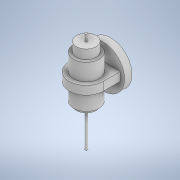
# Autodesk Inventor part: spindle
Saved by Autodesk Inventor 2020 (Build 240168000, 168)
## iProperties
Created: 2021-09-22
Part Number: spindle
Material: Generic
Document SubType Name: Modeling
Designer: zhang
Density: 1 g/cm^3
Appearance: Default
Author: zhang
Autodesk Inventor part; units mm, degrees
ref_plane "YZ Plane" through (0, 0, 0) normal (1, 0, 0) x (0, 1, 0)
ref_plane "XZ Plane" through (0, 0, 0) normal (0, 1, 0) x (-1, 0, 0)
ref_plane "XY Plane" through (0, 0, 0) normal (0, 0, 1) x (1, 0, 0)
sketch "Sketch1" plane through (0, 0, 0) normal (1, 0, 0) x (0, 1, 0)
  line L0 (0, 0) -> (1.5, 2)
  line L1 (1.5, 2) -> (1.5, 43)
  line L2 (0, 59) -> (0, 0)
  line L3 (11.5, 51) -> (16.5, 51)
  line L4 (16.5, 51) -> (16.5, 101)
  line L5 (16.5, 101) -> (11.5, 101)
  line L6 (1.5, 105) -> (1.5, 120)
  line L7 (1.5, 120) -> (0, 120)
  line L8 (0, 120) -> (0, 59)
  line L9 (0, -24) -> (0, 144) projected
  line L10 (16.5, 76) -> (-5.6648, 76)
  line L11 (-30.7978, 0) -> (145.133, 0) projected
  line L12 (11.5, 101) -> (11.5, 105)
  line L13 (11.5, 105) -> (1.5, 105)
  line L14 (11.5, 51) -> (11.5, 47)
  line L15 (11.5, 47) -> (5.5, 47)
  line L16 (5.5, 47) -> (5.5, 43)
  line L17 (5.5, 43) -> (1.5, 43)
  line L18 (0, 0) -> (2, 1.5)
  line L19 (2, 1.5) -> (43, 1.5)
  line L20 (43, 1.5) -> (43, 5.5)
  line L21 (43, 5.5) -> (47, 5.5)
  line L22 (47, 5.5) -> (47, 11.5)
  line L23 (47, 11.5) -> (51, 11.5)
  line L24 (51, 11.5) -> (51, 15)
  line L25 (51, 15) -> (101, 15)
  line L26 (101, 15) -> (101, 11.5)
  line L27 (101, 11.5) -> (112, 11.5)
  line L28 (112, 11.5) -> (112, 1.5)
  line L29 (112, 1.5) -> (120, 1.5)
  line L30 (120, 1.5) -> (120, 0)
  line L31 (-30.7978, 0) -> (145.133, 0) projected
  line L32 (76, 15) -> (76, 0)
  line L33 (0, 0) -> (120, 0)
  dimension "d0" = 2
  dimension "d3" = 76
  dimension "d4" = 120
  dimension "d5" = 50
  dimension "d7" = 1.5
  dimension "d8" = 10
  dimension "d9" = 4
  dimension "d10" = 4
  dimension "d11" = 4
  dimension "d12" = 6
  dimension "d13" = 4
  dimension "d21" = 2
  dimension "d22" = 1.5
  dimension "d23" = 76
  dimension "d24" = 120
  dimension "d25" = 1.5
  dimension "d26" = 4
  dimension "d27" = 4
  dimension "d28" = 6
  dimension "d29" = 4
  dimension "d30" = 10
  dimension "d31" = 8
  dimension "d32" = 50
  dimension "d33" = 15
  dimension "d42" = 3
  constraints: 62 end point, 19 perpendicular, 5 vertical, 3 horizontal, 2 collinear, 2 midpoint, 2 point on line
  measures "d0" vertical distance of L0.start L0.end
  measures "d3" distance between parallel lines of L11 L10
  measures "d4" distance between parallel lines of L11 L7
  measures "d5" diameter of L5 L10
  measures "d7" distance of L6.end L7.end
  measures "d8" distance of L6.start L12.end
  measures "d9" distance of L5.end L12.end
  measures "d10" distance of L3.start L14.end
  measures "d11" distance of L15.end L16.end
  measures "d12" distance of L14.end L15.end
  measures "d13" distance of L1.end L16.end
  measures "d21" horizontal distance of L0.start L18.end
  measures "d22" distance between parallel lines of L31 L19
  measures "d23" distance between parallel lines of L9 L32
  measures "d24" distance from line of L0.start L30
  measures "d25" distance of L29.end L30.end
  measures "d26" distance of L19.end L20.end
  measures "d27" distance of L20.end L21.end
  measures "d28" distance of L21.end L22.end
  measures "d29" distance of L22.end L23.end
  measures "d30" distance of L27.end L28.end
  measures "d31" distance of L28.end L29.end
  measures "d32" distance between parallel lines of L26 L24
  measures "d33" distance between parallel lines of L31 L25
  measures "d42" diameter of L9 L1
revolve "Revolution1" add sketch "Sketch1" angle 360 about axis through (0, -10, 0) along (0, 1, 0) contours L18 L19 L20 L21 L22 L23 L24 L25 L32 L11 | L32 L25 L26 L27 L28 L29 L30 L11
ref_plane "Work Plane2" through (0, 76, 0) normal (0, 1, 0) x (1, 0, 0)
sketch "Sketch4" plane through (0, 76, 0) normal (0, 1, 0) x (1, 0, 0)
  arc A0 (-20, 0) -> (20, 0) centre (0, 0) ccw
  line L0 (-20, 0) -> (-20, 20)
  line L1 (-20, 20) -> (20, 20)
  line L2 (20, 20) -> (20, 0)
  dimension "d35" = 20
  dimension "d36" = 20
  constraints: 6 end point, 3 point on circle, 2 perpendicular, 1 centre point, 1 coincident, 1 vertical
  measures "d35" radius of A0
  measures "d36" distance of L0.start L0.end
extrude "Extrusion3" add sketch "Sketch4" along normal mid plane 10
sketch "Sketch5" plane through (20, 81, -20) normal (0, 0, -1) x (-1, 0, 0)
  line L0 (0, 0) -> (0, -10) projected
  line L1 (0, -5) -> (40, -5) construction
  line L2 (40, -10) -> (40, 0) projected
  circle A0 centre (20, -5) radius 25
  point P0 (20, -81)
  dimension "d39" = 50
  constraints: 3 midpoint, 2 end point, 1 centre point
  measures "d39" diameter of A0
extrude "Extrusion4" add sketch "Sketch5" along normal blind 8.75
body "Solid1"
